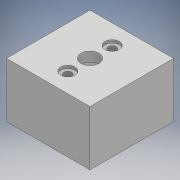
# Autodesk Inventor part: Motor_Support
Saved by Autodesk Inventor 2018.2 (Build 222227000, 227)
## iProperties
Created: 2018-08-11
Part Number: Motor_Support
Material: Generic
Document SubType Name: Modeling
Designer: mateu
Density: 1 g/cm^3
Appearance: Default
Author: mateu
Autodesk Inventor part; units mm, degrees
ref_plane "YZ Plane" through (0, 0, 0) normal (1, 0, 0) x (0, 1, 0)
ref_plane "XZ Plane" through (0, 0, 0) normal (0, 1, 0) x (-1, 0, 0)
ref_plane "XY Plane" through (0, 0, 0) normal (0, 0, 1) x (1, 0, 0)
sketch "Sketch1" plane through (0, 0, 0) normal (0, 0, 1) x (1, 0, 0)
  line L0 (0, 0) -> (35, 0)
  line L1 (35, 0) -> (35, -35)
  line L2 (35, -35) -> (0, -35)
  line L3 (0, -35) -> (0, 0)
  circle A0 centre (17.5, -17.5) radius 12.75
  dimension "d0" = 35
  dimension "d1" = 35
  dimension "d2" = 25.5
  constraints: 8 end point, 2 parallel, 1 centre point, 1 horizontal, 1 perpendicular
  measures "d0" distance of L1.end L2.end
  measures "d1" distance of L0.end L1.end
  measures "d2" diameter of A0
extrude "Extrusion1" add sketch "Sketch1" along normal blind 19
sketch "Sketch2" plane through (0, 0, 19) normal (0, 0, 1) x (1, 0, 0)
  line L0 (35, -35) -> (35, 0) projected
  line L1 (0, 0) -> (35, 0)
  line L2 (35, 0) -> (35, -35)
  line L3 (35, -35) -> (0, -35)
  line L4 (0, -35) -> (0, 0)
  circle A0 centre (17.5, -17.5) radius 3.75
  circle A1 centre (17.5, -8.2) radius 1.65
  circle A2 centre (17.5, -26.8) radius 1.65
  dimension "d5" = 7.5
  dimension "d6" = 17.5
  dimension "d7" = 17.5
  dimension "d8" = 3.3
  dimension "d9" = 3.3
  dimension "d10" = 9.3
  dimension "d11" = 9.3
  constraints: 8 end point, 3 centre point, 2 parallel, 1 horizontal, 1 perpendicular
  measures "d5" diameter of A0
  measures "d6" distance from line of L0 A0.centre
  measures "d7" distance from line of L3 A0.centre
  measures "d8" diameter of A1
  measures "d9" diameter of A2
  measures "d10" distance of A1.centre A0.centre
  measures "d11" distance of A2.centre A0.centre
extrude "Extrusion2" add sketch "Sketch2" along normal blind 4
sketch "Sketch3" plane through (0, 0, 23) normal (0, 0, 1) x (1, 0, 0)
  circle A0 centre (17.5, -8.2) radius 1.65 projected
  circle A1 centre (17.5, -8.2) radius 3
  circle A2 centre (17.5, -26.8) radius 1.65 projected
  circle A3 centre (17.5, -26.8) radius 3
  point P0 (0, 0)
  dimension "d14" = 6
  dimension "d15" = 6
  constraints: 2 centre point, 2 coincident
  measures "d14" diameter of A1
  measures "d15" diameter of A3
extrude "Extrusion3" cut sketch "Sketch3" against normal blind 1.2
body "Solid1"
